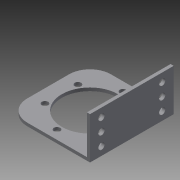
# Autodesk Inventor part: offcenter_L_clamp
Saved by Autodesk Inventor 2015 (Build 190159000, 159)
## iProperties
Created: 2017-09-26
Part Number: offcenter_L_clamp
Material: Generic
Document SubType Name: Modeling
Designer: Anshul
Density: 1 g/cm^3
Appearance: Default
Author: Anshul
Autodesk Inventor part; units mm, degrees
ref_plane "YZ Plane" through (0, 0, 0) normal (1, 0, 0) x (0, 1, 0)
ref_plane "XZ Plane" through (0, 0, 0) normal (0, 1, 0) x (-1, 0, 0)
ref_plane "XY Plane" through (0, 0, 0) normal (0, 0, 1) x (1, 0, 0)
sketch "Sketch1" plane through (0, 0, 0) normal (0, 1, 0) x (-1, 0, 0)
  line L0 (0, 0) -> (0, -40)
  line L1 (0, -40) -> (40, -40)
  line L2 (40, -40) -> (40, 0)
  line L3 (40, 0) -> (0, 0)
  line L4 (0, 0) -> (1.5, 0)
  line L5 (1.5, 0) -> (1.5, -40)
  line L6 (1.5, -40) -> (0, -40)
  circle A0 centre (20, -20) radius 13.5
  circle A1 centre (20, -4.25) radius 1.5
  circle A2 centre (33.6399, -12.125) radius 1.5
  circle A3 centre (33.6399, -27.875) radius 1.5
  circle A4 centre (20, -35.75) radius 1.5
  circle A5 centre (6.3601, -27.875) radius 1.5
  circle A6 centre (6.3601, -12.125) radius 1.5
  dimension "d0" = 40
  dimension "d2" = 1.5
  dimension "d7" = 3
  dimension "d8" = 3
  dimension "d9" = 3
  dimension "d10" = 3
  dimension "d11" = 3
  dimension "d12" = 3
  constraints: 14 end point, 7 centre point, 4 perpendicular, 2 point on line, 1 collinear, 1 vertical
  measures "d0" distance of L0.start L0.end
  measures "d2" distance of L0.start L4.end
  measures "d7" diameter of A1
  measures "d8" diameter of A2
  measures "d9" diameter of A3
  measures "d10" diameter of A4
  measures "d11" diameter of A5
  measures "d12" diameter of A6
extrude "Extrusion1" add sketch "Sketch1" along normal blind 1.5 contours L3 L2 L1 L5
extrude "Extrusion2" add sketch "Sketch1" along normal blind 20 contours L3 L5 L1 L0
sketch "Sketch2" plane through (0, 0, 0) normal (1, 0, 0) x (0, 0, -1)
  line L0 (0, 20) -> (5.5, 20)
  line L1 (0, 20) -> (40, 20) projected
  line L2 (0, 20) -> (34.5, 20)
  line L3 (40, 20) -> (34.5, 20)
  line L4 (34.5, 20) -> (34.5, 16)
  line L5 (34.5, 16) -> (34.5, 10)
  line L6 (34.5, 10) -> (34.5, 4)
  line L7 (5.5, 20) -> (5.5, 16)
  line L8 (5.5, 16) -> (5.5, 10)
  line L9 (5.5, 10) -> (5.5, 4)
  circle A0 centre (5.5, 4) radius 1.5
  circle A1 centre (5.5, 10) radius 1.5
  circle A2 centre (5.5, 16) radius 1.5
  circle A3 centre (34.5, 16) radius 1.5
  circle A4 centre (34.5, 10) radius 1.5
  circle A5 centre (34.5, 4) radius 1.5
  point P0 (0, 0)
  dimension "d17" = 5.5
  dimension "d18" = 34.5
  dimension "d19" = 4
  dimension "d20" = 6
  dimension "d21" = 6
  dimension "d22" = 4
  dimension "d23" = 6
  dimension "d24" = 6
  dimension "d25" = 3
  dimension "d26" = 3
  dimension "d27" = 3
  dimension "d28" = 3
  dimension "d29" = 3
  dimension "d30" = 3
  constraints: 18 end point, 6 centre point, 6 coincident, 6 point on line, 1 collinear, 1 parallel, 1 perpendicular
  measures "d17" distance of L0.start L0.end
  measures "d18" distance of L0.start L2.end
  measures "d19" distance of L2.end L4.end
  measures "d20" distance of L4.end L5.end
  measures "d21" distance of L5.end L6.end
  measures "d22" distance of L0.end L7.end
  measures "d23" distance of L7.end L8.end
  measures "d24" distance of L8.end L9.end
  measures "d25" diameter of A0
  measures "d26" diameter of A1
  measures "d27" diameter of A2
  measures "d28" diameter of A3
  measures "d29" diameter of A4
  measures "d30" diameter of A5
extrude "Extrusion3" cut sketch "Sketch2" against normal blind 5
fillet "Fillet1" radius 10 2 edges at (-40, 0.75, 0) (-40, 0.75, -40)
body "Solid1"
